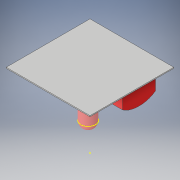
# Autodesk Inventor part: farmer
Saved by Autodesk Inventor 2018 (Build 220112000, 112)
## iProperties
Created: 2018-06-06
Part Number: farmer
Material: Generic
Document SubType Name: Modeling
Designer: 3400746
Density: 1 g/cm^3
Appearance: Default
Author: 3400746
Autodesk Inventor part; units mm, degrees
ref_plane "YZ Plane" through (0, 0, 0) normal (1, 0, 0) x (0, 1, 0)
ref_plane "XZ Plane" through (0, 0, 0) normal (0, 1, 0) x (-1, 0, 0)
sketch "Sketch1" plane through (0, 0, 0) normal (0, 1, 0) x (-1, 0, 0)
  line L0 (0, 0) -> (2159, 0)
  line L1 (2159, 0) -> (2159, -2159)
  line L2 (2159, -2159) -> (0, -2159)
  line L3 (0, -2159) -> (0, 0)
  dimension "d0" = 2159
  dimension "d1" = 2159
  dimension "d2" = 2159
  dimension "d3" = 2159
  constraints: 8 end point, 2 perpendicular, 1 horizontal
  measures "d0" distance of L0.start L0.end
  measures "d1" distance of L0.end L1.end
  measures "d2" distance of L1.end L2.end
  measures "d3" distance of L2.end L0.start
extrude "Extrusion1" add sketch "Sketch1" along normal blind 25.4
sketch "Sketch3" plane through (0, 0, 0) normal (0, -1, 0) x (1, 0, 0)
  line L0 (0, 0) -> (0, -2159) projected
  line L1 (0, -2159) -> (0, -1079.5)
  line L2 (0, -1079.5) -> (-241.3, -1079.5)
  line L3 (-241.3, -1079.5) -> (-241.3, -1930.4)
  line L4 (-241.3, -1930.4) -> (-1003.3, -1930.4)
  line L5 (-1003.3, -1930.4) -> (-1003.3, -1079.5)
  line L6 (-241.3, -1079.5) -> (-1003.3, -1079.5)
  dimension "d6" = 241.3
  dimension "d7" = 850.9
  dimension "d8" = 762
  dimension "d9" = 850.9
  constraints: 12 end point, 2 perpendicular, 1 horizontal, 1 midpoint, 1 vertical
  measures "d6" distance of L1.end L2.end
  measures "d7" distance of L2.end L3.end
  measures "d8" distance of L3.end L4.end
  measures "d9" distance of L4.end L5.end
extrude "Extrusion2" add sketch "Sketch3" along normal blind 508
sketch "Sketch4" plane through (-1003.3, 0, -1930.4) normal (-1, 0, 0) x (0, 0, 1)
  line L0 (0, 0) -> (0, -508) projected
  line L1 (0, -508) -> (425.45, -508)
  line L2 (0, -508) -> (850.9, -508) projected
  line L3 (425.45, -508) -> (425.45, -635)
  arc A0 (0, -508) -> (425.45, -635) centre (402.3685, 63.8059) ccw
  arc A1 (425.45, -635) -> (850.9, -508) centre (440.9735, 89.1252) ccw
  point P0 (1930.4, 0)
  dimension "d12" = 425.45
  dimension "d13" = 127
  constraints: 4 end point, 4 point on circle, 2 centre point, 1 midpoint, 1 perpendicular
  measures "d12" distance of L0.end L1.end
  measures "d13" distance of L1.end L3.end
extrude "Extrusion3" add sketch "Sketch4" against normal blind 762
sketch "Sketch5" plane through (-1003.3, 0, -1930.4) normal (-1, 0, 0) x (0, 0, 1)
  line L0 (0, 0) -> (0, -508) projected
  line L1 (0, 0) -> (425.45, 0)
  line L2 (0, 0) -> (850.9, 0) projected
  line L3 (425.45, 0) -> (425.45, -203.2)
  line L4 (425.45, -203.2) -> (298.45, -203.2)
  line L5 (298.45, -203.2) -> (298.45, 0)
  line L6 (425.45, -203.2) -> (552.45, -203.2)
  line L7 (552.45, -203.2) -> (552.45, 0)
  line L8 (552.45, 0) -> (425.45, 0)
  line L9 (425.45, -203.2) -> (438.15, -203.2)
  line L10 (438.15, -190.5) -> (539.75, -190.5)
  line L11 (539.75, -190.5) -> (539.75, -12.7)
  line L12 (539.75, -12.7) -> (438.15, -12.7)
  line L13 (438.15, -12.7) -> (438.15, -190.5)
  line L14 (412.75, -190.5) -> (311.15, -190.5)
  line L15 (311.15, -190.5) -> (311.15, -12.7)
  line L16 (311.15, -12.7) -> (412.75, -12.7)
  line L17 (412.75, -12.7) -> (412.75, -190.5)
  point P0 (1930.4, 0)
  dimension "d16" = 425.45
  dimension "d17" = 203.2
  dimension "d18" = 127
  dimension "d19" = 127
  dimension "d20" = 203.2
  dimension "d23" = 101.6
  dimension "d24" = 177.8
  dimension "d25" = 101.6
  dimension "d27" = 101.6
  dimension "d28" = 177.8
  dimension "d29" = 101.6
  dimension "d30" = 177.8
  constraints: 32 end point, 4 perpendicular, 4 point on line, 1 collinear, 1 horizontal, 1 midpoint, 1 parallel, 1 vertical
  measures "d16" distance of L0.start L1.end
  measures "d17" distance of L1.end L3.end
  measures "d18" distance of L3.end L4.end
  measures "d19" distance of L3.end L6.end
  measures "d20" distance of L6.end L7.end
  measures "d23" distance of L10.start L10.end
  measures "d24" distance of L10.end L11.end
  measures "d25" distance of L11.end L12.end
  measures "d27" distance of L14.start L14.end
  measures "d28" distance of L14.end L15.end
  measures "d29" distance of L15.end L16.end
  measures "d30" distance of L16.end L14.start
extrude "Extrusion4" add sketch "Sketch5" along normal blind 2.54
sketch "Sketch6" plane through (-1003.3, -190.5, -1492.25) normal (-1, 0, 0) x (0, 0, 1)
  line L0 (0, 0) -> (101.6, 0) projected
  line L1 (101.6, 0) -> (93.98, 0)
  line L2 (101.6, 177.8) -> (0, 177.8) projected
  line L3 (0, 177.8) -> (0, 170.18)
  line L4 (0, 177.8) -> (0, 0) projected
  line L5 (0, 170.18) -> (93.98, 0)
  line L6 (101.6, 177.8) -> (101.6, 0) projected
  line L7 (101.6, 0) -> (101.6, 7.62)
  line L8 (0, 177.8) -> (7.62, 177.8)
  line L9 (7.62, 177.8) -> (101.6, 7.62)
  line L10 (0, 0) -> (7.62, 0)
  line L11 (0, 0) -> (0, 7.62)
  line L12 (101.6, 177.8) -> (93.98, 177.8)
  line L13 (101.6, 177.8) -> (101.6, 170.18)
  line L14 (93.98, 177.8) -> (50.8, 99.6092)
  line L15 (44.886, 88.9) -> (0, 7.62)
  line L16 (7.62, 0) -> (50.8, 78.1908)
  line L17 (56.714, 88.9) -> (101.6, 170.18)
  line L18 (-25.4, 0) -> (-127, 0) projected
  line L19 (-25.4, 0) -> (-33.02, 0)
  line L20 (-25.4, 0) -> (-25.4, 7.62)
  line L21 (-25.4, 0) -> (-25.4, 177.8) projected
  line L22 (-127, 176.3789) -> (-127, 168.7589)
  line L23 (-127, 177.8) -> (-127, 0) projected
  line L24 (-127, 177.8) -> (-119.38, 177.8)
  line L25 (-127, 177.8) -> (-25.4, 177.8) projected
  line L26 (-127, 0) -> (-127, 7.62)
  line L27 (-127, 0) -> (-119.38, 0)
  line L28 (-25.4, 177.8) -> (-25.4, 170.18)
  line L29 (-25.4, 177.8) -> (-33.02, 177.8)
  line L30 (-33.02, 177.8) -> (-127, 7.62)
  line L31 (-119.38, 0) -> (-25.4, 170.18)
  line L32 (-127, 168.7589) -> (-82.3199, 88.5273)
  line L33 (-76.381, 77.863) -> (-33.02, 0)
  line L34 (-76.2, 99.6092) -> (-119.38, 177.8)
  line L35 (-70.286, 88.9) -> (-25.4, 7.62)
  point P0 (1492.25, 190.5)
  dimension "d33" = 7.62
  dimension "d34" = 7.62
  dimension "d35" = 7.62
  dimension "d36" = 7.62
  dimension "d37" = 7.62
  dimension "d38" = 7.62
  dimension "d39" = 7.62
  dimension "d40" = 7.62
  dimension "d41" = 7.62
  dimension "d42" = 7.62
  dimension "d43" = 7.62
  dimension "d44" = 7.62
  constraints: 56 end point, 24 point on line
  measures "d33" distance of L0.end L1.end
  measures "d34" distance of L2.end L3.end
  measures "d35" distance of L0.end L7.end
  measures "d36" distance of L2.end L8.end
  measures "d37" distance of L0.start L11.end
  measures "d38" distance of L18.start L19.end
  measures "d39" distance of L18.start L20.end
  measures "d40" distance of L22.start L22.end
  measures "d41" distance of L23.start L24.end
  measures "d42" distance of L18.end L27.end
  measures "d43" distance of L21.end L28.end
  measures "d44" distance of L21.end L29.end
extrude "Extrusion5" add sketch "Sketch6" along normal blind 2.54 contours L4 L15 L5 L16 L0 | L5 L3 L2 L9 L6 L0 | L17 L9 L14 L2 L6 | L18 L33 L31 L35 L20 | L18 L23 L30 L25 L21 L31 | L22 L23 L24 L34 L30 L32
sketch "Sketch7" plane through (0, 0, 0) normal (0, -1, 0) x (1, 0, 0)
  line L0 (0, -2159) -> (0, 0) projected
  line L1 (0, 0) -> (0, -711.2)
  line L2 (0, -711.2) -> (-762, -711.2)
  circle A0 centre (-762, -711.2) radius 190.5
  dimension "d47" = 711.2
  dimension "d48" = 762
  dimension "d49" = 381
  constraints: 4 end point, 1 centre point, 1 coincident, 1 perpendicular, 1 point on line
  measures "d47" distance of L0.end L1.end
  measures "d48" distance of L1.end L2.end
  measures "d49" diameter of A0
extrude "Extrusion6" add sketch "Sketch7" along normal blind 812.8
sketch "Sketch8" plane through (-762, -812.8, -711.2) normal (0, -1, 0) x (1, 0, 0)
  line L0 (0, 0) -> (0, -190.5)
  circle A0 centre (0, 0) radius 190.5 projected
  point P0 (762, 711.2)
  constraints: 2 end point, 1 vertical, 1 vertical alignment, 1 other
ref_plane "Work Plane1" through (-762, -812.8, -711.2) normal (-1, 0, 0) x (0, 0, -1)
sketch "Sketch9" plane through (-762, -812.8, -711.2) normal (-1, 0, 0) x (0, 0, -1)
  line L0 (190.5, 0) -> (-190.5, 0) projected
  line L1 (0, 0) -> (0, 177.8)
  arc A0 (190.5, 0) -> (0, 177.8) centre (4.6676, -8.1525) ccw
  arc A1 (0, 177.8) -> (-190.5, 0) centre (13.9606, -28.1113) ccw
  point P0 (-711.2, -812.8)
  dimension "d53" = 177.8
  constraints: 4 point on circle, 2 centre point, 2 end point, 1 midpoint, 1 vertical
  measures "d53" distance of L1.start L1.end
revolve "Revolution1" add sketch "Sketch9" angle 360 about axis through (-762, -812.8, -711.2) along (0, -1, 0) contours L0 L1 A0
sketch "Sketch10" plane through (0, 0, 0) normal (0, -1, 0) x (1, 0, 0)
  line L0 (-2159, 0) -> (-2159, -2159) projected
  line L1 (-2159, 0) -> (-1905, 0)
  line L2 (-2159, 0) -> (0, 0) projected
  line L3 (-1905, 0) -> (-1905, -254)
  line L4 (-1905, -254) -> (-1270, -254)
  line L5 (-1270, -254) -> (-1270, -1397)
  line L6 (-1270, -1397) -> (-1905, -1397)
  line L7 (-1905, -1397) -> (-1905, -254)
  dimension "d55" = 254
  dimension "d56" = 254
  dimension "d57" = 635
  dimension "d59" = 1143
  dimension "d60" = 635
  constraints: 12 end point, 3 perpendicular, 1 point on line, 1 vertical
  measures "d55" distance of L0.start L1.end
  measures "d56" distance of L1.end L3.end
  measures "d57" distance of L3.end L4.end
  measures "d59" distance of L4.end L5.end
  measures "d60" distance of L5.end L6.end
extrude "Extrusion7" add sketch "Sketch10" along normal blind 2.54
sketch "Sketch11" plane through (0, -2.54, 0) normal (0, -1, 0) x (1, 0, 0)
  line L0 (-1270, -254) -> (-1905, -254) projected
  line L1 (-1270, -254) -> (-1270, -381)
  line L2 (-1270, -381) -> (-1270, -508)
  line L3 (-1270, -1397) -> (-1270, -254) projected
  line L4 (-1270, -508) -> (-1270, -635)
  line L5 (-1270, -635) -> (-1270, -762)
  line L6 (-1270, -762) -> (-1270, -889)
  line L7 (-1270, -889) -> (-1270, -1016)
  line L8 (-1270, -1016) -> (-1270, -1143)
  line L9 (-1270, -1143) -> (-1270, -1270)
  line L10 (-1270, -1270) -> (-1270, -1397)
  line L11 (-1270, -381) -> (-1905, -381)
  line L12 (-1270, -508) -> (-1905, -508)
  line L13 (-1905, -254) -> (-1905, -1397) projected
  line L14 (-1270, -635) -> (-1905, -635)
  line L15 (-1270, -762) -> (-1905, -762)
  line L16 (-1270, -889) -> (-1905, -889)
  line L17 (-1270, -1016) -> (-1905, -1016)
  line L18 (-1270, -1143) -> (-1905, -1143)
  line L19 (-1270, -1270) -> (-1905, -1270)
  line L20 (-1270, -254) -> (-1397, -254)
  line L21 (-1397, -254) -> (-1397, -1397)
  line L22 (-1397, -254) -> (-1524, -254)
  line L23 (-1524, -254) -> (-1524, -1397)
  line L24 (-1524, -254) -> (-1651, -254)
  line L25 (-1651, -254) -> (-1778, -254)
  line L26 (-1778, -254) -> (-1905, -254)
  line L27 (-1651, -254) -> (-1651, -1397)
  line L28 (-1778, -254) -> (-1778, -1397)
  circle A0 centre (-1397, -381) radius 6.35
  circle A1 centre (-1397, -508) radius 6.35
  circle A2 centre (-1397, -635) radius 6.35
  circle A3 centre (-1397, -762) radius 6.35
  circle A4 centre (-1397, -889) radius 6.35
  circle A5 centre (-1397, -1016) radius 6.35
  circle A6 centre (-1397, -1143) radius 6.35
  circle A7 centre (-1397, -1270) radius 6.35
  circle A8 centre (-1524, -1270) radius 6.35
  circle A9 centre (-1651, -1270) radius 6.35
  circle A10 centre (-1778, -1270) radius 6.35
  circle A11 centre (-1778, -1143) radius 6.35
  circle A12 centre (-1778, -1016) radius 6.35
  circle A13 centre (-1778, -889) radius 6.35
  circle A14 centre (-1778, -762) radius 6.35
  circle A15 centre (-1778, -635) radius 6.35
  circle A16 centre (-1778, -508) radius 6.35
  circle A17 centre (-1778, -381) radius 6.35
  circle A18 centre (-1651, -381) radius 6.35
  circle A19 centre (-1524, -381) radius 6.35
  circle A20 centre (-1524, -508) radius 6.35
  circle A21 centre (-1651, -508) radius 6.35
  circle A22 centre (-1524, -635) radius 6.35
  circle A23 centre (-1651, -635) radius 6.35
  circle A24 centre (-1524, -762) radius 6.35
  circle A25 centre (-1651, -762) radius 6.35
  circle A26 centre (-1524, -889) radius 6.35
  circle A27 centre (-1524, -1016) radius 6.35
  circle A28 centre (-1651, -889) radius 6.35
  circle A29 centre (-1651, -1016) radius 6.35
  circle A30 centre (-1524, -1143) radius 6.35
  circle A31 centre (-1651, -1143) radius 6.35
  point P0 (0, 0)
  dimension "d63" = 127
  dimension "d66" = 127
  dimension "d67" = 127
  dimension "d68" = 127
  dimension "d69" = 127
  dimension "d70" = 127
  dimension "d71" = 127
  dimension "d72" = 127
  dimension "d73" = 127
  dimension "d74" = 127
  dimension "d75" = 127
  dimension "d77" = 1143
  dimension "d78" = 127
  dimension "d79" = 127
  dimension "d80" = 127
  dimension "d81" = 1143
  dimension "d82" = 1143
  dimension "d83" = 12.7
  dimension "d84" = 12.7
  dimension "d85" = 12.7
  dimension "d86" = 12.7
  dimension "d87" = 12.7
  dimension "d88" = 12.7
  dimension "d89" = 12.7
  dimension "d90" = 12.7
  dimension "d91" = 12.7
  dimension "d92" = 12.7
  dimension "d93" = 12.7
  dimension "d94" = 12.7
  dimension "d95" = 12.7
  dimension "d96" = 12.7
  dimension "d97" = 12.7
  dimension "d98" = 12.7
  dimension "d99" = 12.7
  dimension "d100" = 12.7
  dimension "d101" = 12.7
  dimension "d102" = 12.7
  dimension "d103" = 12.7
  dimension "d104" = 12.7
  dimension "d105" = 12.7
  dimension "d106" = 12.7
  dimension "d107" = 12.7
  dimension "d108" = 12.7
  dimension "d109" = 12.7
  dimension "d110" = 12.7
  dimension "d111" = 12.7
  dimension "d112" = 12.7
  dimension "d113" = 12.7
  dimension "d114" = 12.7
  constraints: 44 end point, 36 point on line, 32 centre point, 11 horizontal, 2 collinear, 60 other
  measures "d63" distance of L0.start L1.end
  measures "d66" distance of L1.end L2.end
  measures "d67" distance of L2.end L4.end
  measures "d68" distance of L4.end L5.end
  measures "d69" distance of L5.end L6.end
  measures "d70" distance of L6.end L7.end
  measures "d71" distance of L7.end L8.end
  measures "d72" distance of L8.end L9.end
  measures "d73" distance of L9.end L10.end
  measures "d74" distance of L0.start L20.end
  measures "d75" distance of L20.end L22.end
  measures "d77" distance of L22.end point (-1524, -1397)
  measures "d78" distance of L22.end L24.end
  measures "d79" distance of L24.end L25.end
  measures "d80" distance of L25.end L0.end
  measures "d81" distance of L24.end point (-1651, -1397)
  measures "d82" distance of L25.end point (-1778, -1397)
  measures "d83" diameter of A0
  measures "d84" diameter of A1
  measures "d85" diameter of A2
  measures "d86" diameter of A3
  measures "d87" diameter of A4
  measures "d88" diameter of A5
  measures "d89" diameter of A6
  measures "d90" diameter of A7
  measures "d91" diameter of A8
  measures "d92" diameter of A9
  measures "d93" diameter of A10
  measures "d94" diameter of A11
  measures "d95" diameter of A12
  measures "d96" diameter of A13
  measures "d97" diameter of A14
  measures "d98" diameter of A15
  measures "d99" diameter of A16
  measures "d100" diameter of A17
  measures "d101" diameter of A18
  measures "d102" diameter of A19
  measures "d103" diameter of A20
  measures "d104" diameter of A21
  measures "d105" diameter of A22
  measures "d106" diameter of A23
  measures "d107" diameter of A24
  measures "d108" diameter of A25
  measures "d109" diameter of A26
  measures "d110" diameter of A27
  measures "d111" diameter of A28
  measures "d112" diameter of A29
  measures "d113" diameter of A30
  measures "d114" diameter of A31
extrude "Extrusion8" add sketch "Sketch11" along normal blind 76.2 contours A0 L11 L21 | L21 L11 A0 | A0 L21 L11 | A19 L11 L23 | L23 L11 A19 | L21 A0 L11 | A1 L21 L12 | L12 L21 A1 | A18 L11 L27 | L27 L11 A18 | L23 A19 L11 | L11 A19 L23 | A2 L21 L14 | L14 L21 A2 | L21 A1 L12 | L12 A1 L21 | A17 L11 L28 | L28 L11 A17 | L27 A18 L11 | L11 A18 L27 | A3 L21 L15 | L15 L21 A3 | L21 A2 L14 | L14 A2 L21 | L28 A17 L11 | L11 A17 L28 | A20 L12 L23 | L23 L12 A20 | A4 L21 L16 | L16 L21 A4 | L21 A3 L15 | L15 A3 L21 | A20 L23 L12 | A21 L12 L27 | L27 L12 A21 | L23 A20 L12 | A5 L21 L17 | L17 L21 A5 | L21 A4 L16 | L16 A4 L21 | A22 L23 L14 | L14 L23 A22 | A16 L28 L12 | L12 L28 A16 | A16 L12 L28 | L27 A21 L12 | L12 A21 L27 | A6 L21 L18 | L18 L21 A6 | L21 A5 L17 | L17 A5 L21 | A24 L23 L15 | L15 L23 A24 | L23 A22 L14 | L14 A22 L23 | L12 A16 L28 | A15 L28 L14 | L14 L28 A15 | A7 L21 L19 | L19 L21 A7 | L21 A6 L18 | L18 A6 L21 | A26 L23 L16 | L16 L23 A26 | L23 A24 L15 | L15 A24 L23 | A15 L14 L28 | A14 L28 L15 | L15 L28 A14 | L14 A15 L28 | A23 L14 L27 | L27 L14 A23 | L21 A7 L19 | L19 A7 L21 | A27 L23 L17 | L17 L23 A27 | L23 A26 L16 | L16 A26 L23 | A23 L27 L14 | A13 L28 L16 | L16 L28 A13 | L28 A14 L15 | L15 A14 L28 | L27 A23 L14 | A30 L23 L18 | L18 L23 A30 | L23 A27 L17 | L17 A27 L23 | A25 L27 L15 | L15 L27 A25 | A12 L28 L17 | L17 L28 A12 | L28 A13 L16 | L16 A13 L28 | A8 L23 L19 | L19 L23 A8 | L23 A30 L18 | L18 A30 L23 | A28 L27 L16 | L16 L27 A28 | L27 A25 L15 | L15 A25 L27 | A11 L28 L18 | L18 L28 A11 | L28 A12 L17 | L17 A12 L28 | L23 A8 L19 | L19 A8 L23 | A29 L27 L17 | L17 L27 A29 | L27 A28 L16 | L16 A28 L27 | A10 L28 L19 | L19 L28 A10 | L28 A11 L18 | L18 A11 L28 | A31 L27 L18 | L18 L27 A31 | L27 A29 L17 | L17 A29 L27 | L28 A10 L19 | L19 A10 L28 | A9 L27 L19 | L19 L27 A9 | L27 A31 L18 | L18 A31 L27 | L27 A9 L19 | L19 A9 L27
body "Solid1"
